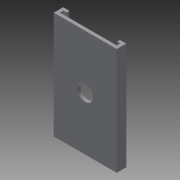
# Autodesk Inventor part: arm-slot
Saved by Autodesk Inventor 2015 (Build 190159000, 159)
## iProperties
Created: 2014-07-18
Part Number: arm-slot
Material: Generic
Document SubType Name: Modeling
Designer: pc
Density: 1 g/cm^3
Appearance: Default
Author: pc
Autodesk Inventor part; units mm, degrees
ref_plane "YZ Plane" through (0, 0, 0) normal (1, 0, 0) x (0, 1, 0)
ref_plane "XZ Plane" through (0, 0, 0) normal (0, 1, 0) x (-1, 0, 0)
ref_plane "XY Plane" through (0, 0, 0) normal (0, 0, 1) x (1, 0, 0)
sketch "Sketch1" plane through (0, 0, 0) normal (0, 1, 0) x (-1, 0, 0)
  line L0 (9.98, 16.98) -> (-9.98, 16.98)
  line L1 (-9.98, 16.98) -> (-9.98, -16.98)
  line L2 (-9.98, -16.98) -> (9.98, -16.98)
  line L3 (9.98, -16.98) -> (9.98, 16.98)
  line L4 (9.98, 16.98) -> (-9.98, -16.98) construction
  line L5 (-9.98, 16.98) -> (9.98, -16.98) construction
  point P0 (0, 0)
  dimension "d0" = 33.96
  dimension "d1" = 19.96
  constraints: 12 end point, 2 midpoint, 2 parallel, 1 horizontal, 1 perpendicular
  measures "d0" distance of L0.end L1.end
  measures "d1" distance of L0.start L0.end
extrude "arm-wall" add sketch "Sketch1" along normal blind 3
sketch "Sketch2" plane through (0, 3, 0) normal (0, 1, 0) x (1, 0, 0)
  line L0 (-8, -16.98) -> (8, -16.98)
  line L1 (8, -16.98) -> (8, 15.98)
  line L2 (8, 15.98) -> (-8, 15.98)
  line L3 (-8, 15.98) -> (-8, -16.98)
  line L4 (-8, -16.98) -> (8, 15.98) construction
  line L5 (8, -16.98) -> (-8, 15.98) construction
  line L6 (0, 23.772) -> (0, -23.772) projected
  line L7 (9.98, 16.98) -> (-9.98, 16.98) projected
  line L8 (-9.98, -16.98) -> (9.98, -16.98) projected
  point P0 (0, 0)
  point P1 (0, -0.5)
  point P2 (0, -0.5)
  dimension "d4" = 16
  dimension "d5" = 1
  constraints: 12 end point, 3 midpoint, 2 parallel, 1 collinear, 1 horizontal, 1 perpendicular, 1 point on line
  measures "d4" distance of L1.end L2.end
  measures "d5" distance between parallel lines of L7 L2
extrude "slot" cut sketch "Sketch2" against normal blind 2
sketch "Sketch3" plane through (0, 0, 0) normal (0, -1, 0) x (1, 0, 0)
  circle A0 centre (0, 0) radius 2.5
  dimension "d12" = 5
  constraints: 1 centre point, 1 coincident
  measures "d12" diameter of A0
extrude "Extrusion3" cut sketch "Sketch3" against normal blind 2
sketch "Sketch4" plane through (-9.98, 0, 16.98) normal (0, 0, 1) x (1, 0, 0)
  line L0 (1.98, 1) -> (0.98, 1)
  line L1 (0.98, 1) -> (0.98, 2.1)
  line L2 (0.98, 2.1) -> (1.98, 2.1)
  line L3 (1.98, 2.1) -> (1.98, 1)
  line L4 (17.98, 1) -> (18.98, 1)
  line L5 (18.98, 1) -> (18.98, 2.1)
  line L6 (18.98, 2.1) -> (17.98, 2.1)
  line L7 (17.98, 2.1) -> (17.98, 1)
  point P0 (9.98, 0)
  dimension "d15" = 1
  dimension "d16" = 1.1
  dimension "d17" = 1
  dimension "d18" = 1.1
  constraints: 16 end point, 4 parallel, 2 horizontal, 2 perpendicular
  measures "d15" distance of L1.end L2.end
  measures "d16" distance of L0.end L1.end
  measures "d17" distance of L6.end L5.end
  measures "d18" distance of L5.end L4.end
extrude "Extrusion4" cut sketch "Sketch4" against normal up to surface (32.96 mm away)
equation "\"d2\" = armthick"
equation "\"d4\" = adapterh"
equation "\"d5\" = -0.5 * adapterw + 0.5 * armw"
equation "\"d6\" = armslotd"
equation "\"d18\" = d16"
equation "\"printer3dtolerance\" = 0.12"
equation "\"wallw\" = 42"
equation "\"wallh\" = 44"
equation "\"cornerrad\" = 2"
equation "\"baseextra\" = 2"
equation "\"wall1_thick\" = 8"
equation "\"wall2_thick\" = 6.4"
equation "\"wall3_thick\" = 4"
equation "\"wall1slot\" = 8.12"
equation "\"wall2slot\" = 6.52"
equation "\"wall3slot\" = 4.12"
equation "\"gap2\" = 28"
equation "\"baseh\" = 79.12"
equation "\"basew\" = 44"
equation "\"base_thick\" = 6"
equation "\"base_slots_depth\" = 4"
equation "\"servobigcircledia\" = 11.62"
equation "\"servosmallcircledia\" = 5.92"
equation "\"servo9gw\" = 22.8"
equation "\"servomounth\" = 4"
equation "\"servomountsquare\" = 4"
equation "\"servopolygonr\" = 6.12"
equation "\"servopolygonl\" = 5.92"
equation "\"distancefrombottom\" = 34"
equation "\"distancefromleft\" = 22"
equation "\"wall3slotd\" = 2"
equation "\"wall3slotw\" = 36"
equation "\"adapterh\" = 16"
equation "\"adapterw\" = 32"
equation "\"armw\" = 34"
equation "\"armslotd\" = 2"
equation "\"armthick\" = 3"
equation "\"fanhb\" = 11"
equation "\"fanhs\" = 9.6"
equation "\"adapterwallslotd\" = 2"
equation "\"adapterwallthick\" = 6"
equation "\"armhornthick\" = 3"
equation "\"hornscrewholed\" = 2"
equation "\"hornscrewheadd\" = 3"
equation "\"hornthick\" = 1.5"
body "Solid1"
